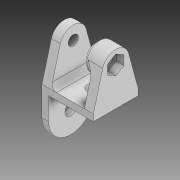
# Autodesk Inventor part: ZIdler
Saved by Autodesk Inventor 2020 (Build 240168000, 168)
## iProperties
Created: 2020-10-21
Part Number: ZIdler
Material: Generic
Document SubType Name: Modeling
Designer: DDeGo
Density: 1 g/cm^3
Appearance: Default
Author: DDeGo
Autodesk Inventor part; units mm, degrees
ref_plane "YZ Plane" through (0, 0, 0) normal (1, 0, 0) x (0, 1, 0)
ref_plane "XZ Plane" through (0, 0, 0) normal (0, 1, 0) x (-1, 0, 0)
sketch "Sketch1" plane through (0, 0, 0) normal (0, 0, 1) x (1, 0, 0)
  line L0 (0, 0) -> (23, 0)
  line L1 (23, 0) -> (23, -3)
  line L2 (23, -3) -> (3, -3)
  line L3 (3, -3) -> (3, -23)
  line L4 (3, -23) -> (0, -23)
  line L5 (0, -23) -> (0, 0)
  dimension "d0" = 3
  dimension "d1" = 20
  constraints: 12 end point, 7 perpendicular, 1 horizontal
  measures "d0" distance of L0.end L1.end
  measures "d1" distance of L1.end L2.end
extrude "Extrusion1" add sketch "Sketch1" along normal mid plane 20
sketch "Sketch2" plane through (0, 0, 10) normal (0, 1, 0) x (1, 0, 0)
  line L0 (23, 20) -> (23, 0) projected
  line L1 (23, 10) -> (13, 10) construction
  circle A0 centre (13, 10) radius 2.75
  line L2 (3, 20) -> (3, 0) projected
  dimension "d14" = 10
  dimension "d15" = 5.5
  constraints: 2 end point, 1 centre point, 1 coincident, 1 horizontal, 1 midpoint
  measures "d14" distance from line of L2 L1.end
  measures "d15" diameter of A0
extrude "Extrusion2" cut sketch "Sketch2" against normal through all
sketch "Sketch3" plane through (0, -23, 10) normal (-1, 0, 0) x (0, 0, 1)
  line L0 (-20, 0) -> (0, 0) projected
  line L1 (-10, 0) -> (-10, 10) construction
  circle A0 centre (-10, 10) radius 2.75
  line L2 (-20, 20) -> (0, 20) projected
  point P0 (-10, 23)
  dimension "d10" = 10
  dimension "d11" = 5.5
  constraints: 2 end point, 1 centre point, 1 coincident, 1 midpoint, 1 vertical
  measures "d10" distance from line of L1.end L2
  measures "d11" diameter of A0
extrude "Extrusion3" cut sketch "Sketch3" against normal through all
sketch "Sketch5" plane through (0, -23, 10) normal (-1, 0, 0) x (0, 0, 1)
  line L0 (-10, 23) -> (-10, 37) construction
  arc A0 (-4.207908, 38.56578) -> (-15.792092, 38.56578) centre (-10, 37) ccw
  circle A1 centre (-10, 37) radius 2.25
  line L1 (-20, 23) -> (0, 23)
  line L2 (-20, 23) -> (-15.792092, 38.56578)
  line L3 (-4.207908, 38.56578) -> (0, 23)
  line L4 (0, 23) -> (-20, 23)
  circle A2 centre (-10, 37) radius 9 construction
  line L5 (-5.857187, 28) -> (-14.47006, 28) construction
  dimension "d23" = 4.5
  dimension "d24" = 12
  dimension "d25" = 14
  dimension "d44" = 18
  dimension "d45" = 5
  constraints: 10 end point, 3 centre point, 3 coincident, 2 point on circle, 2 tangent, 1 collinear, 1 horizontal, 1 vertical
  measures "d23" diameter of A1
  measures "d24" diameter of A0
  measures "d25" distance of L0.start L0.end
  measures "d44" diameter of A2
  measures "d45" distance between parallel lines of L1 L5
extrude "Extrusion5" add sketch "Sketch5" against normal blind 4
sketch "Sketch6" plane through (23, -3, 10) normal (1, 0, 0) x (0, 0, -1)
  line L0 (4.207908, 18.56578) -> (0, 3)
  line L1 (20, 3) -> (0, 3)
  line L2 (20, 3) -> (15.792092, 18.56578)
  arc A0 (15.792092, 18.56578) -> (4.207908, 18.56578) centre (10, 17) ccw
  circle A1 centre (10, 17) radius 2.25
  point P0 (10, 3)
extrude "Extrusion6" add sketch "Sketch6" against normal blind 4
fillet "Fillet1" radius 10 2 edges at (1.5, -23, 10) (1.5, -23, -10)
ref_plane "Work Plane2" through (14, -23, 10) normal (1, 0, 0) x (0, 0, -1)
sketch "Sketch7" plane through (19, -3, 10) normal (-1, 0, 0) x (0, 0, 1)
  circle A0 centre (-10, 17) radius 2.25
  arc A1 (-4.207908, 18.56578) -> (-15.792092, 18.56578) centre (-10, 17) ccw
  circle A2 centre (-10, 17) radius 6
  point P0 (-10, 3)
  point P1 (-15.792092, 18.56578)
  constraints: 1 coincident, 3 other
extrude "Extrusion7" add sketch "Sketch7" along normal up to surface (5 mm away)
sketch "Sketch8" plane through (23, -3, 10) normal (1, 0, 0) x (0, 0, -1)
  circle A0 centre (10, 17) radius 2.25
  line L0 (10, 21.214657) -> (13.65, 19.107328)
  line L1 (13.65, 19.107328) -> (13.65, 14.892672)
  line L2 (13.65, 14.892672) -> (10, 12.785343)
  line L3 (10, 12.785343) -> (6.35, 14.892672)
  line L4 (6.35, 14.892672) -> (6.35, 19.107328)
  line L5 (6.35, 19.107328) -> (10, 21.214657)
  point P0 (10, 3)
  dimension "d37" = 7.3
  constraints: 12 end point, 1 coincident, 1 vertical, 13 other
  measures "d37" distance between parallel lines of L1 L4
extrude "Extrusion8" cut sketch "Sketch8" against normal blind 3.5 contours A0 | L0 L1 L2 L3 L4 L5
chamfer "Chamfer2" distance 2 angle 45 2 edges at (14, 8, 0) (14, 20, 0)
fillet "Fillet2" radius 2.5 2 edges at (19, 8, 0) (4, 0, 0)
body "Solid1"
